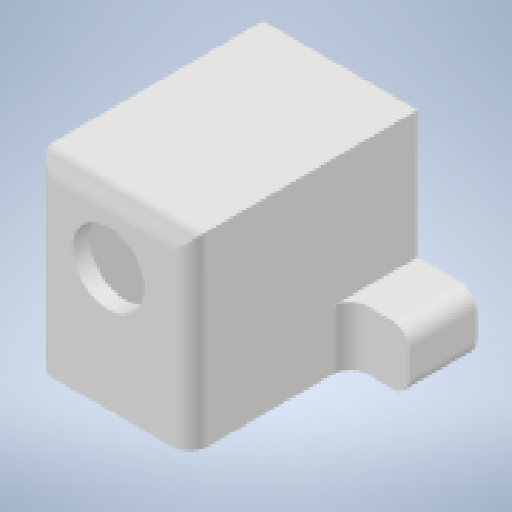
# Autodesk Inventor part: fast_switch
Saved by Autodesk Inventor 2023 (Build 270158000, 158)
## iProperties
Created: 2026-02-26
Part Number: fast_switch
Material: Типовые
Document SubType Name: Modeling
Designer: garin
Density: 1 g/cm^3
Appearance: По умолчанию
Author: garin
Autodesk Inventor part; units mm, degrees
ref_plane "YZ Plane" through (0, 0, 0) normal (1, 0, 0) x (0, 1, 0)
ref_plane "XZ Plane" through (0, 0, 0) normal (0, 1, 0) x (-1, 0, 0)
ref_plane "XY Plane" through (0, 0, 0) normal (0, 0, 1) x (1, 0, 0)
sketch "Эскиз1" plane through (0, 0, 0) normal (0, 0, 1) x (1, 0, 0)
  line L0 (0, 0) -> (-38, 0) construction
  line L1 (-38, 0) -> (-38, 25) construction
  line L2 (-38, 25) -> (0, 25) construction
  line L3 (0, 25) -> (0, 0) construction
  line L4 (-38, 25) -> (-35, 25) construction
  line L5 (-35, 25) -> (-35, 23.5) construction
  line L6 (-35, 23.5) -> (-38, 23.5) construction
  line L7 (-38, 23.5) -> (-38, 25) construction
  line L8 (-35, 23.5) -> (-23.7, 23.5)
  line L9 (-23.7, 23.5) -> (-23.7, 3.2)
  line L10 (-23.7, 3.2) -> (-35, 3.2)
  line L11 (-35, 3.2) -> (-35, 23.5)
  line L12 (-35, 25) -> (-35, 25.3) construction
  line L13 (-35, 25.3) -> (-38, 25.3) construction
  line L14 (-35, 23.5) -> (-36, 23.5) construction
  line L15 (-36, 23.5) -> (-36, 24.5) construction
  line L16 (-36, 24.5) -> (-35, 24.5) construction
  line L17 (-35, 24.5) -> (-35, 23.5) construction
  line L18 (-36, 24.5) -> (-22.7, 24.5)
  line L19 (-22.7, 24.5) -> (-22.7, 3.2)
  line L20 (-22.7, 3.2) -> (-36, 3.2)
  line L21 (-36, 3.2) -> (-36, 24.5)
  line L22 (-38, 25.3) -> (-19.7, 25.3)
  line L23 (-19.7, 25.3) -> (-19.7, 3.2)
  line L24 (-19.7, 3.2) -> (-38, 3.2)
  line L25 (-38, 3.2) -> (-38, 25.3)
  line L26 (-23.7, 23.5) -> (-35, 23.5) construction
  line L27 (-35, 23.5) -> (-35, 17.74) construction
  line L28 (-35, 17.74) -> (-23.7, 17.74) construction
  line L29 (-23.7, 17.74) -> (-23.7, 23.5) construction
  circle A0 centre (-29.35, 17.74) radius 4.25
  line L30 (-19.7, 3.2) -> (-12.7, 3.2)
  line L31 (-12.7, 3.2) -> (-12.7, 10.2)
  line L32 (-12.7, 10.2) -> (-19.7, 10.2)
  line L33 (-19.7, 10.2) -> (-19.7, 3.2)
  line L34 (-16.2, 10.2) -> (-16.2, 3.2) construction
  line L35 (-12.7, 6.7) -> (-19.7, 6.7) construction
  circle A1 centre (-16.2, 6.7) radius 2.1
  line L36 (-29.35, 17.74) -> (-29.35, 18.74)
  point P0 (-23.7, 3.2)
  dimension "d0" = 38
  dimension "d1" = 25
  dimension "d2" = 3
  dimension "d3" = 1.5
  dimension "d4" = 11.3
  dimension "d5" = 20.3
  dimension "d6" = 0.3
  dimension "d7" = 1
  dimension "d8" = 1
  dimension "d9" = 13.3
  dimension "d10" = 21.3
  dimension "d11" = 18.3
  dimension "d12" = 5.76
  dimension "d13" = 8.5
  dimension "d19" = 7
  dimension "d20" = 7
  dimension "d21" = 4.2
  dimension "d27" = 1
  constraints: 74 end point, 16 parallel, 11 perpendicular, 8 horizontal, 6 midpoint, 2 centre point, 1 point on line
  measures "d0" distance of L1.end L2.end
  measures "d1" distance of L0.end L1.end
  measures "d2" distance of L5.end L6.end
  measures "d3" distance of L4.end L5.end
  measures "d4" distance of L9.end L10.end
  measures "d5" distance of L8.end L9.end
  measures "d6" distance of L4.end L12.end
  measures "d7" distance of L15.end L16.end
  measures "d8" distance of L14.end L15.end
  measures "d9" distance of L19.end L20.end
  measures "d10" distance of L18.end L19.end
  measures "d11" distance of L23.end L24.end
  measures "d12" distance of L27.end L26.end
  measures "d13" diameter of A0
  measures "d19" distance of L32.end L31.end
  measures "d20" distance of L31.end L30.end
  measures "d21" diameter of A1
  measures "d27" distance of L36.start L36.end
extrude "Выдавливание1" add sketch "Эскиз1" along normal blind 27 contours L24 L25 L22 L23 L19 L18 L21
extrude "Выдавливание2" add sketch "Эскиз1" against normal blind 2 from surface at 27 contours L11 L20 L21 L18 L19 L9 L8 | L8 L9 L10 L11
fillet "Сопряжение1" radius 2 3 edges at (-38, 14.25, 27) (-28.85, 25.3, 27) (-19.7, 14.25, 27)
extrude "Выдавливание3" add sketch "Эскиз1" along normal blind 8 contours L23 L32 L31 L30 | A1
extrude "Выдавливание4" cut sketch "Эскиз1" along normal blind 6 contours A1
fillet "Сопряжение2" radius 2 3 edges at (-12.7, 10.2, 4) (-12.7, 3.2, 4) (-19.7, 6.7, 8)
